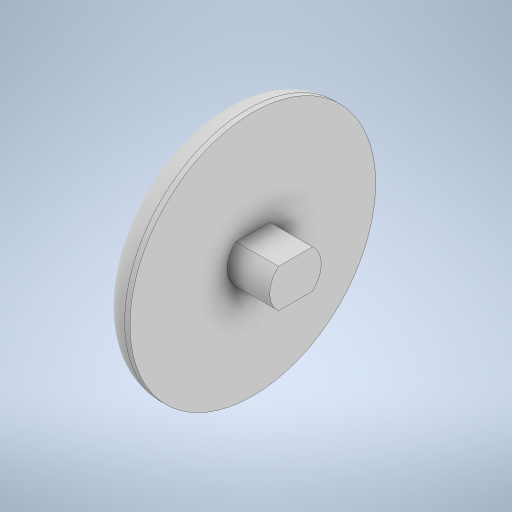
# Autodesk Inventor part: cap
Saved by Autodesk Inventor 2023 (Build 270158000, 158)
## iProperties
Created: 2025-12-21
Part Number: cap
Material: Generic
Document SubType Name: Modeling
Designer: Justin Pascual
Density: 1 g/cm^3
Appearance: Default
Author: Justin Pascual
Autodesk Inventor part; units mm, degrees
ref_plane "YZ Plane" through (0, 0, 0) normal (1, 0, 0) x (0, 1, 0)
ref_plane "XZ Plane" through (0, 0, 0) normal (0, 1, 0) x (-1, 0, 0)
ref_plane "XY Plane" through (0, 0, 0) normal (0, 0, 1) x (1, 0, 0)
sketch "Sketch1" plane through (0, 0, 0) normal (1, 0, 0) x (0, 1, 0)
  circle A0 centre (0, 0) radius 14.605
  dimension "d0" = 29.21
  constraints: 1 centre point, 1 coincident
  measures "d0" diameter of A0
extrude "Extrusion1" add sketch "Sketch1" along normal blind 3.81
sketch "Sketch2" plane through (3.81, 0, 0) normal (1, 0, 0) x (0, 0, -1)
  circle A0 centre (0, 0) radius 3.048
  dimension "d3" = 6.096
  constraints: 1 centre point, 1 coincident
  measures "d3" diameter of A0
extrude "Extrusion2" add sketch "Sketch2" along normal blind 5.08
fillet "Fillet1" radius 3.175 1 edges at (0, -14.605, 0)
sketch "Sketch4" plane through (0, 0, 0) normal (-1, 0, 0) x (0, 0, 1)
  arc A0 (-5.6465, -0.0713) -> (-5.6554, -0.2762) centre (-3.74, -0.2569) ccw
  arc A1 (-5.6141, 0.1942) -> (-5.6465, -0.0713) centre (-0.2253, -0.5991) ccw
  arc A2 (-5.5662, 0.4727) -> (-5.6141, 0.1942) centre (0.1529, -0.6547) ccw
  arc A3 (-5.5086, 0.7215) -> (-5.5662, 0.4727) centre (-1.7406, -0.2815) ccw
  arc A4 (-5.4267, 0.9766) -> (-5.5086, 0.7215) centre (-2.9409, 0.038) ccw
  arc A5 (-5.304, 1.2751) -> (-5.4267, 0.9766) centre (-0.2248, -0.9874) ccw
  arc A6 (-5.163, 1.5684) -> (-5.304, 1.2751) centre (-0.1685, -1.0125) ccw
  arc A7 (-5.0245, 1.8082) -> (-5.163, 1.5684) centre (-2.5323, 0.209) ccw
  arc A8 (-4.869, 2.0358) -> (-5.0245, 1.8082) centre (-1.0123, -0.7664) ccw
  arc A9 (-4.676, 2.2913) -> (-4.869, 2.0358) centre (2.1392, -3.0561) ccw
  arc A10 (-4.4775, 2.535) -> (-4.676, 2.2913) centre (1.9807, -2.9319) ccw
  arc A11 (-4.3056, 2.7244) -> (-4.4775, 2.535) centre (-1.6197, 0.1159) ccw
  arc A12 (-4.1196, 2.9069) -> (-4.3056, 2.7244) centre (-0.4386, -1.0312) ccw
  arc A13 (-3.8757, 3.1295) -> (-4.1196, 2.9069) centre (5.2583, -7.1259) ccw
  arc A14 (-3.6172, 3.3542) -> (-3.8757, 3.1295) centre (5.6741, -7.5927) ccw
  arc A15 (-3.384, 3.5453) -> (-3.6172, 3.3542) centre (1.9777, -3.2377) ccw
  arc A16 (-3.1278, 3.7362) -> (-3.384, 3.5453) centre (0.0717, -0.8264) ccw
  arc A17 (-2.7957, 3.9619) -> (-3.1278, 3.7362) centre (4.7659, -7.5206) ccw
  arc A18 (-2.4462, 4.1848) -> (-2.7957, 3.9619) centre (5.0689, -7.9808) ccw
  arc A19 (-2.1334, 4.3689) -> (-2.4462, 4.1848) centre (1.9799, -2.9802) ccw
  arc A20 (-1.7942, 4.5471) -> (-2.1334, 4.3689) centre (1.421, -1.9817) ccw
  arc A21 (-1.3601, 4.7537) -> (-1.7942, 4.5471) centre (6.0902, -11.4629) ccw
  arc A22 (-0.9069, 4.9546) -> (-1.3601, 4.7537) centre (6.3782, -12.0897) ccw
  arc A23 (-0.5051, 5.1169) -> (-0.9069, 4.9546) centre (3.3555, -5.0178) ccw
  arc A24 (-0.5051, 5.1169) -> (-0.1633, 5.2508) centre (-7.5686, 23.6598) ccw
  arc A25 (-0.1633, 5.2508) -> (0.1029, 5.3637) centre (-3.0503, 12.4277) ccw
  arc A26 (0.1029, 5.3637) -> (0.2863, 5.4497) centre (-2.0951, 10.2878) ccw
  arc A27 (0.2863, 5.4497) -> (0.2822, 5.4684) centre (0.282, 5.4585) ccw
  arc A28 (1.732, 5.7393) -> (1.7288, 5.6986) centre (1.7542, 5.7171) ccw
  arc A29 (1.7288, 5.6986) -> (1.8415, 5.5509) centre (5.1977, 8.2289) ccw
  arc A30 (1.8415, 5.5509) -> (1.9924, 5.3743) centre (4.5398, 7.7039) ccw
  arc A31 (1.9924, 5.3743) -> (2.1821, 5.1752) centre (6.9782, 9.9337) ccw
  arc A32 (2.4175, 4.9127) -> (2.1821, 5.1752) centre (-0.2932, 2.7193) ccw
  arc A33 (2.6207, 4.6321) -> (2.4175, 4.9127) centre (-0.1096, 2.8679) ccw
  arc A34 (2.791, 4.3346) -> (2.6207, 4.6321) centre (-0.0502, 2.9062) ccw
  arc A35 (2.9276, 4.0215) -> (2.791, 4.3346) centre (-0.0136, 2.9247) ccw
  arc A36 (3.0322, 3.7206) -> (2.9276, 4.0215) centre (-3.7608, 1.5272) ccw
  arc A37 (3.1484, 3.3453) -> (3.0322, 3.7206) centre (-12.5502, -1.3107) ccw
  arc A38 (3.2578, 2.9596) -> (3.1484, 3.3453) centre (-12.9445, -1.4276) ccw
  arc A39 (3.3418, 2.6247) -> (3.2578, 2.9596) centre (-5.6824, 0.5388) ccw
  arc A40 (3.4241, 2.1569) -> (3.3418, 2.6247) centre (-1.0267, 1.615) ccw
  arc A41 (3.4758, 1.5875) -> (3.4241, 2.1569) centre (-5.844, 1.0284) ccw
  arc A42 (3.5034, 0.8484) -> (3.4758, 1.5875) centre (-12.8805, 0.6063) ccw
  arc A43 (3.5094, -0.1688) -> (3.5034, 0.8484) centre (-53.4811, 0.0065) ccw
  arc A44 (3.4966, -1.3751) -> (3.5094, -0.1688) centre (-76.6004, 0.0774) ccw
  arc A45 (3.459, -2.053) -> (3.4966, -1.3751) centre (-5.6132, -1.2099) ccw
  arc A46 (3.3775, -2.6038) -> (3.459, -2.053) centre (-1.657, -1.5776) ccw
  arc A47 (3.2212, -3.2698) -> (3.3775, -2.6038) centre (-7.9955, -0.2856) ccw
  arc A48 (3.093, -3.71) -> (3.2212, -3.2698) centre (-6.2812, -0.7417) ccw
  arc A49 (2.941, -4.1565) -> (3.093, -3.71) centre (-7.3983, -0.3879) ccw
  arc A50 (2.7884, -4.5487) -> (2.941, -4.1565) centre (-6.23, -0.8138) ccw
  arc A51 (2.6634, -4.8003) -> (2.7884, -4.5487) centre (0.8989, -3.7662) ccw
  arc A52 (2.5346, -4.9925) -> (2.6634, -4.8003) centre (1.0054, -3.8286) ccw
  arc A53 (2.3759, -5.1807) -> (2.5346, -4.9925) centre (0.576, -3.5018) ccw
  arc A54 (2.2126, -5.3386) -> (2.3759, -5.1807) centre (0.7613, -3.6747) ccw
  arc A55 (2.0722, -5.4341) -> (2.2126, -5.3386) centre (1.7464, -4.8041) ccw
  arc A56 (1.8649, -5.5155) -> (2.0722, -5.4341) centre (1.5744, -4.4716) ccw
  arc A57 (1.6748, -5.5367) -> (1.8649, -5.5155) centre (1.7045, -4.939) ccw
  arc A58 (1.419, -5.5007) -> (1.6748, -5.5367) centre (1.746, -4.103) ccw
  arc A59 (0.9213, -5.3769) -> (1.419, -5.5007) centre (5.6118, 12.4168) ccw
  arc A60 (0.5621, -5.28) -> (0.9213, -5.3769) centre (9.1798, 25.9517) ccw
  arc A61 (0.1735, -5.1709) -> (0.5621, -5.28) centre (12.4982, 37.9783) ccw
  arc A62 (-0.1873, -5.0661) -> (0.1735, -5.1709) centre (11.5162, 34.5399) ccw
  arc A63 (-0.4514, -4.9848) -> (-0.1873, -5.0661) centre (3.3268, 6.8259) ccw
  arc A64 (-0.7227, -4.8868) -> (-0.4514, -4.9848) centre (0.738, -1.2668) ccw
  arc A65 (-1.1143, -4.7232) -> (-0.7227, -4.8868) centre (5.8148, 11.3157) ccw
  arc A66 (-1.5449, -4.531) -> (-1.1143, -4.7232) centre (6.6251, 13.1912) ccw
  arc A67 (-1.9539, -4.3357) -> (-1.5449, -4.531) centre (5.4282, 10.5949) ccw
  arc A68 (-2.372, -4.1184) -> (-1.9539, -4.3357) centre (3.2302, 6.1494) ccw
  arc A69 (-2.8306, -3.8595) -> (-2.372, -4.1184) centre (6.3574, 11.881) ccw
  arc A70 (-3.2602, -3.6002) -> (-2.8306, -3.8595) centre (5.8348, 10.9857) ccw
  arc A71 (-3.5828, -3.3849) -> (-3.2602, -3.6002) centre (0.0383, 1.6898) ccw
  arc A72 (-3.873, -3.1625) -> (-3.5828, -3.3849) centre (-0.4693, 0.9784) ccw
  arc A73 (-4.197, -2.8843) -> (-3.873, -3.1625) centre (2.4433, 4.5218) ccw
  arc A74 (-4.5043, -2.5966) -> (-4.197, -2.8843) centre (2.3234, 4.388) ccw
  arc A75 (-4.7417, -2.3458) -> (-4.5043, -2.5966) centre (-1.3894, 0.5899) ccw
  arc A76 (-4.9465, -2.0901) -> (-4.7417, -2.3458) centre (-1.9464, 0.1021) ccw
  arc A77 (-5.1523, -1.7887) -> (-4.9465, -2.0901) centre (-0.3352, 1.2794) ccw
  arc A78 (-5.3296, -1.4893) -> (-5.1523, -1.7887) centre (-0.6214, 1.0972) ccw
  arc A79 (-5.444, -1.2432) -> (-5.3296, -1.4893) centre (-3.5575, -0.5158) ccw
  arc A80 (-5.5236, -1.0061) -> (-5.444, -1.2432) centre (-2.7878, -0.2191) ccw
  arc A81 (-5.5915, -0.7375) -> (-5.5236, -1.0061) centre (-1.4164, 0.1755) ccw
  arc A82 (-5.6392, -0.479) -> (-5.5915, -0.7375) centre (-1.6866, 0.1164) ccw
  arc A83 (-5.6554, -0.2762) -> (-5.6392, -0.479) centre (-4.1953, -0.2615) ccw
  arc A84 (-0.8061, 0.9371) -> (-0.8024, 0.86) centre (-0.6453, 0.9061) ccw
  arc A85 (-0.8024, 0.86) -> (-0.7642, 0.7759) centre (-0.4887, 0.952) ccw
  arc A86 (-0.7642, 0.7759) -> (-0.6987, 0.6978) centre (-0.4301, 0.9895) ccw
  arc A87 (-0.6987, 0.6978) -> (-0.6152, 0.6385) centre (-0.4234, 0.9967) ccw
  arc A88 (-0.6152, 0.6385) -> (-0.5006, 0.591) centre (-0.3178, 1.1941) ccw
  arc A89 (-0.5006, 0.591) -> (-0.3373, 0.5486) centre (0.1071, 2.5958) ccw
  arc A90 (-0.3373, 0.5486) -> (-0.1569, 0.5168) centre (0.1561, 2.8218) ccw
  arc A91 (-0.1569, 0.5168) -> (0.0144, 0.5018) centre (0.0865, 2.3088) ccw
  arc A92 (0.0144, 0.5018) -> (0.1943, 0.5059) centre (0.0714, 1.9317) ccw
  arc A93 (0.1943, 0.5059) -> (0.401, 0.5323) centre (-0.0258, 3.0602) ccw
  arc A94 (0.401, 0.5323) -> (0.6017, 0.5747) centre (-0.017, 3.0079) ccw
  arc A95 (0.6017, 0.5747) -> (0.7626, 0.6281) centre (0.3107, 1.7191) ccw
  arc A96 (0.7626, 0.6281) -> (0.8943, 0.6933) centre (0.3445, 1.6375) ccw
  arc A97 (0.8943, 0.6933) -> (1.0055, 0.7714) centre (0.4905, 1.3868) ccw
  arc A98 (1.0055, 0.7714) -> (1.0832, 0.8503) centre (0.6344, 1.2148) ccw
  arc A99 (1.0832, 0.8503) -> (1.1065, 0.9159) centre (1.0024, 0.9159) ccw
  arc A100 (1.1065, 0.9159) -> (1.0851, 0.983) centre (0.9908, 0.9159) ccw
  arc A101 (1.0851, 0.983) -> (1.0134, 1.0668) centre (0.5836, 0.6263) ccw
  arc A102 (1.0134, 1.0668) -> (0.9109, 1.1518) centre (0.4374, 0.4764) ccw
  arc A103 (0.9109, 1.1518) -> (0.7895, 1.2252) centre (0.3037, 0.2856) ccw
  arc A104 (0.7895, 1.2252) -> (0.6424, 1.2879) centre (0.2947, 0.2683) ccw
  arc A105 (0.6424, 1.2879) -> (0.4615, 1.3405) centre (-0.0227, -0.6623) ccw
  arc A106 (0.4615, 1.3405) -> (0.2768, 1.3763) centre (-0.0219, -0.659) ccw
  arc A107 (0.2768, 1.3763) -> (0.118, 1.3876) centre (0.1228, 0.3266) ccw
  arc A108 (0.118, 1.3876) -> (-0.0373, 1.3771) centre (0.1236, 0.148) ccw
  arc A109 (-0.0373, 1.3771) -> (-0.211, 1.3467) centre (0.227, -0.6422) ccw
  arc A110 (-0.211, 1.3467) -> (-0.3762, 1.3026) centre (0.2088, -0.5599) ccw
  arc A111 (-0.3762, 1.3026) -> (-0.5042, 1.2506) centre (-0.1235, 0.4982) ccw
  arc A112 (-0.5042, 1.2506) -> (-0.6091, 1.1856) centre (-0.1798, 0.6096) ccw
  arc A113 (-0.6091, 1.1856) -> (-0.7033, 1.1026) centre (-0.1505, 0.5703) ccw
  arc A114 (-0.7033, 1.1026) -> (-0.774, 1.015) centre (-0.2392, 0.6557) ccw
  arc A115 (-0.774, 1.015) -> (-0.8061, 0.9371) centre (-0.5985, 0.8971) ccw
  arc A116 (-0.702, 0.9022) -> (-0.72, 0.8615) centre (-0.665, 0.8615) ccw
  arc A117 (-0.6411, 0.9476) -> (-0.702, 0.9022) centre (-0.4441, 0.6193) ccw
  arc A118 (-0.5542, 0.99) -> (-0.6411, 0.9476) centre (-0.35, 0.4625) ccw
  arc A119 (-0.4514, 1.0227) -> (-0.5542, 0.99) centre (-0.2383, 0.1739) ccw
  arc A120 (-0.329, 1.0437) -> (-0.4514, 1.0227) centre (-0.2529, 0.2319) ccw
  arc A121 (-0.1828, 1.0505) -> (-0.329, 1.0437) centre (-0.1828, -0.5159) ccw
  arc A122 (-0.0365, 1.0437) -> (-0.1828, 1.0505) centre (-0.1828, -0.5159) ccw
  arc A123 (0.0858, 1.0227) -> (-0.0365, 1.0437) centre (-0.1127, 0.2319) ccw
  arc A124 (0.1887, 0.99) -> (0.0858, 1.0227) centre (-0.1272, 0.1739) ccw
  arc A125 (0.2755, 0.9476) -> (0.1887, 0.99) centre (-0.0155, 0.4625) ccw
  arc A126 (0.3365, 0.9022) -> (0.2755, 0.9476) centre (0.0786, 0.6193) ccw
  arc A127 (0.3544, 0.8615) -> (0.3365, 0.9022) centre (0.2994, 0.8615) ccw
  arc A128 (0.3365, 0.8209) -> (0.3544, 0.8615) centre (0.2994, 0.8615) ccw
  arc A129 (0.2755, 0.7755) -> (0.3365, 0.8209) centre (0.0786, 1.1038) ccw
  arc A130 (0.1887, 0.7331) -> (0.2755, 0.7755) centre (-0.0155, 1.2606) ccw
  arc A131 (0.0858, 0.7004) -> (0.1887, 0.7331) centre (-0.1272, 1.5491) ccw
  arc A132 (-0.0365, 0.6794) -> (0.0858, 0.7004) centre (-0.1127, 1.4912) ccw
  arc A133 (-0.1828, 0.6726) -> (-0.0365, 0.6794) centre (-0.1828, 2.2389) ccw
  arc A134 (-0.329, 0.6794) -> (-0.1828, 0.6726) centre (-0.1828, 2.2389) ccw
  arc A135 (-0.4514, 0.7004) -> (-0.329, 0.6794) centre (-0.2529, 1.4912) ccw
  arc A136 (-0.5542, 0.7331) -> (-0.4514, 0.7004) centre (-0.2384, 1.5491) ccw
  arc A137 (-0.6411, 0.7755) -> (-0.5542, 0.7331) centre (-0.35, 1.2606) ccw
  arc A138 (-0.702, 0.8209) -> (-0.6411, 0.7755) centre (-0.4441, 1.1038) ccw
  arc A139 (-0.72, 0.8615) -> (-0.702, 0.8209) centre (-0.665, 0.8615) ccw
  arc A140 (1.1654, 2.4636) -> (1.1531, 2.1926) centre (3.902, 2.2035) ccw
  arc A141 (1.1531, 2.1926) -> (1.1654, 1.8953) centre (5.1247, 2.2083) ccw
  arc A142 (1.1654, 1.8953) -> (1.1993, 1.6066) centre (4.9828, 2.1971) ccw
  arc A143 (1.1993, 1.6066) -> (1.2524, 1.3622) centre (3.2813, 1.9315) ccw
  arc A144 (1.2524, 1.3622) -> (1.3214, 1.1513) centre (3.7833, 2.0724) ccw
  arc A145 (1.3214, 1.1513) -> (1.41, 0.9394) centre (4.14, 2.2059) ccw
  arc A146 (1.41, 0.9394) -> (1.504, 0.7559) centre (3.8105, 2.053) ccw
  arc A147 (1.504, 0.7559) -> (1.5876, 0.6397) centre (2.0638, 1.0707) ccw
  arc A148 (1.5876, 0.6397) -> (1.6762, 0.5537) centre (2.2968, 1.2815) ccw
  arc A149 (1.6762, 0.5537) -> (1.7836, 0.4708) centre (2.5832, 1.6174) ccw
  arc A150 (1.7836, 0.4708) -> (1.8928, 0.4024) centre (2.5272, 1.5371) ccw
  arc A151 (1.8928, 0.4024) -> (1.9855, 0.3623) centre (2.1366, 0.8385) ccw
  arc A152 (1.9855, 0.3623) -> (2.0826, 0.3491) centre (2.072, 0.6348) ccw
  arc A153 (2.0826, 0.3491) -> (2.2048, 0.3645) centre (2.0567, 1.0462) ccw
  arc A154 (2.2048, 0.3645) -> (2.3315, 0.4035) centre (2.0379, 1.1326) ccw
  arc A155 (2.3315, 0.4035) -> (2.4429, 0.4617) centre (2.0932, 0.9953) ccw
  arc A156 (2.4429, 0.4617) -> (2.5515, 0.5599) centre (2.1836, 0.8575) ccw
  arc A157 (2.5515, 0.5599) -> (2.6713, 0.7272) centre (1.1834, 1.6661) ccw
  arc A158 (2.6713, 0.7272) -> (2.7826, 0.9278) centre (0.9458, 1.8161) ccw
  arc A159 (2.7826, 0.9278) -> (2.8674, 1.1344) centre (1.1347, 1.7247) ccw
  arc A160 (2.8674, 1.1344) -> (2.9338, 1.3723) centre (0.7866, 1.8433) ccw
  arc A161 (2.9338, 1.3723) -> (2.9896, 1.6702) centre (-1.8893, 2.4304) ccw
  arc A162 (2.9896, 1.6702) -> (3.0279, 1.9773) centre (-2.0236, 2.4514) ccw
  arc A163 (3.0279, 1.9773) -> (3.0405, 2.2451) centre (0.1745, 2.2451) ccw
  arc A164 (3.0405, 2.2451) -> (3.0258, 2.5429) centre (0.0074, 2.2451) ccw
  arc A165 (3.0258, 2.5429) -> (2.9818, 2.8162) centre (0.7805, 2.3213) ccw
  arc A166 (2.9818, 2.8162) -> (2.9066, 3.0728) centre (0.9388, 2.3569) ccw
  arc A167 (2.9066, 3.0728) -> (2.7987, 3.3204) centre (0.8572, 2.3272) ccw
  arc A168 (2.7987, 3.3204) -> (2.6928, 3.5094) centre (0.2659, 2.0248) ccw
  arc A169 (2.6928, 3.5094) -> (2.5744, 3.6865) centre (0.4245, 2.1217) ccw
  arc A170 (2.5744, 3.6865) -> (2.4606, 3.8304) centre (0.7326, 2.346) ccw
  arc A171 (2.4606, 3.8304) -> (2.3746, 3.9031) centre (2.1908, 3.5987) ccw
  arc A172 (2.3746, 3.9031) -> (2.2771, 3.9441) centre (2.1862, 3.5911) ccw
  arc A173 (2.2771, 3.9441) -> (2.1648, 3.9591) centre (2.1579, 3.4811) ccw
  arc A174 (2.1648, 3.9591) -> (2.0389, 3.9477) centre (2.1561, 3.355) ccw
  arc A175 (2.0389, 3.9477) -> (1.9013, 3.9099) centre (2.2286, 2.9881) ccw
  arc A176 (1.9013, 3.9099) -> (1.7746, 3.8431) centre (2.0686, 3.4386) ccw
  arc A177 (1.7746, 3.8431) -> (1.6383, 3.7275) centre (2.4729, 2.8824) ccw
  arc A178 (1.6383, 3.7275) -> (1.5124, 3.5837) centre (2.568, 2.7861) ccw
  arc A179 (1.5124, 3.5837) -> (1.4159, 3.4306) centre (2.3632, 2.9409) ccw
  arc A180 (1.4159, 3.4306) -> (1.3373, 3.2447) centre (2.5829, 2.8273) ccw
  arc A181 (1.3373, 3.2447) -> (1.2621, 2.9914) centre (4.9275, 2.0417) ccw
  arc A182 (1.2621, 2.9914) -> (1.2011, 2.7174) centre (5.2222, 1.9653) ccw
  arc A183 (1.2011, 2.7174) -> (1.1654, 2.4636) centre (3.9974, 2.1944) ccw
  arc A184 (1.2182, 2.3502) -> (1.214, 2.2129) centre (3.4297, 2.2129) ccw
  arc A185 (1.2313, 2.4658) -> (1.2182, 2.3502) centre (2.364, 2.279) ccw
  arc A186 (1.2499, 2.5531) -> (1.2313, 2.4658) centre (2.1922, 2.3074) ccw
  arc A187 (1.273, 2.571) -> (1.2499, 2.5531) centre (1.273, 2.5471) ccw
  arc A188 (1.3103, 2.5638) -> (1.273, 2.571) centre (1.273, 2.4713) ccw
  arc A189 (1.4079, 2.5229) -> (1.3103, 2.5638) centre (-0.1186, -0.979) ccw
  arc A190 (1.5234, 2.4699) -> (1.4079, 2.5229) centre (0.0725, -0.5406) ccw
  arc A191 (1.6491, 2.4071) -> (1.5234, 2.4699) centre (-0.6443, -2.0277) ccw
  arc A192 (1.7704, 2.3386) -> (1.6491, 2.4071) centre (0.7674, 0.7022) ccw
  arc A193 (1.8727, 2.2685) -> (1.7704, 2.3386) centre (1.139, 1.3083) ccw
  arc A194 (1.9485, 2.2046) -> (1.8727, 2.2685) centre (1.2448, 1.4468) ccw
  arc A195 (1.9654, 2.1653) -> (1.9485, 2.2046) centre (1.9124, 2.1658) ccw
  arc A196 (1.9483, 2.1254) -> (1.9654, 2.1653) centre (1.9089, 2.1658) ccw
  arc A197 (1.8728, 2.058) -> (1.9483, 2.1254) centre (1.1542, 2.9393) ccw
  arc A198 (1.7714, 1.9832) -> (1.8728, 2.058) centre (1.0535, 3.0629) ccw
  arc A199 (1.6513, 1.9092) -> (1.7714, 1.9832) centre (0.6483, 3.6722) ccw
  arc A200 (1.5267, 1.8454) -> (1.6513, 1.9092) centre (0.8629, 3.295) ccw
  arc A201 (1.4117, 1.8015) -> (1.5267, 1.8454) centre (1.1283, 2.7154) ccw
  arc A202 (1.3184, 1.7792) -> (1.4117, 1.8015) centre (1.1989, 2.4876) ccw
  arc A203 (1.2759, 1.7928) -> (1.3184, 1.7792) centre (1.3103, 1.8272) ccw
  arc A204 (1.2517, 1.8367) -> (1.2759, 1.7928) centre (1.3396, 1.8565) ccw
  arc A205 (1.2322, 1.9417) -> (1.2517, 1.8367) centre (2.6334, 2.1483) ccw
  arc A206 (1.2185, 2.0712) -> (1.2322, 1.9417) centre (2.7946, 2.1721) ccw
  arc A207 (1.214, 2.2129) -> (1.2185, 2.0712) centre (3.4321, 2.2129) ccw
  arc A208 (1.3479, 1.4473) -> (1.3282, 1.416) centre (1.3588, 1.4186) ccw
  arc A209 (1.4339, 1.4729) -> (1.3479, 1.4473) centre (1.5622, 0.8849) ccw
  arc A210 (1.5538, 1.4908) -> (1.4339, 1.4729) centre (1.6269, 0.5885) ccw
  arc A211 (1.6975, 1.4966) -> (1.5538, 1.4908) centre (1.6975, -0.2825) ccw
  arc A212 (1.8532, 1.4879) -> (1.6975, 1.4966) centre (1.6975, 0.1) ccw
  arc A213 (1.9712, 1.4604) -> (1.8532, 1.4879) centre (1.7954, 0.973) ccw
  arc A214 (2.0452, 1.4176) -> (1.9712, 1.4604) centre (1.8895, 1.2339) ccw
  arc A215 (2.0699, 1.3623) -> (2.0452, 1.4176) centre (1.9999, 1.3642) ccw
  arc A216 (2.0548, 1.2939) -> (2.0699, 1.3623) centre (1.8855, 1.3672) ccw
  arc A217 (2.0045, 1.192) -> (2.0548, 1.2939) centre (0.9985, 1.7514) ccw
  arc A218 (1.9345, 1.0793) -> (2.0045, 1.192) centre (0.8064, 1.8582) ccw
  arc A219 (1.8524, 0.971) -> (1.9345, 1.0793) centre (0.6931, 1.9365) ccw
  arc A220 (1.767, 0.8758) -> (1.8524, 0.971) centre (0.5068, 2.0916) ccw
  arc A221 (1.6877, 0.8031) -> (1.767, 0.8758) centre (1.1305, 1.4899) ccw
  arc A222 (1.6223, 0.7566) -> (1.6877, 0.8031) centre (1.2912, 1.2918) ccw
  arc A223 (1.5923, 0.7601) -> (1.6223, 0.7566) centre (1.6095, 0.7773) ccw
  arc A224 (1.5689, 0.7918) -> (1.5923, 0.7601) centre (1.6869, 0.8547) ccw
  arc A225 (1.5288, 0.8703) -> (1.5689, 0.7918) centre (3.7941, 1.9761) ccw
  arc A226 (1.4845, 0.966) -> (1.5288, 0.8703) centre (3.8278, 1.9926) ccw
  arc A227 (1.4407, 1.0708) -> (1.4845, 0.966) centre (4.6256, 2.3421) ccw
  arc A228 (1.3997, 1.178) -> (1.4407, 1.0708) centre (4.9842, 2.4853) ccw
  arc A229 (1.3641, 1.2814) -> (1.3997, 1.178) centre (4.3502, 2.254) ccw
  arc A230 (1.3368, 1.3697) -> (1.3641, 1.2814) centre (4.14, 2.1856) ccw
  arc A231 (1.3282, 1.416) -> (1.3368, 1.3697) centre (1.5646, 1.436) ccw
  arc A232 (1.4946, 3.3391) -> (1.445, 3.2157) centre (2.7811, 2.7499) ccw
  arc A233 (1.551, 3.4433) -> (1.4946, 3.3391) centre (2.3051, 2.9679) ccw
  arc A234 (1.6061, 3.5185) -> (1.551, 3.4433) centre (2.1144, 3.0881) ccw
  arc A235 (1.6482, 3.538) -> (1.6061, 3.5185) centre (1.6482, 3.4829) ccw
  arc A236 (1.6936, 3.5234) -> (1.6482, 3.538) centre (1.6482, 3.46) ccw
  arc A237 (1.761, 3.4685) -> (1.6936, 3.5234) centre (1.2818, 2.9488) ccw
  arc A238 (1.8345, 3.3921) -> (1.761, 3.4685) centre (1.1591, 2.8158) ccw
  arc A239 (1.9046, 3.3016) -> (1.8345, 3.3921) centre (0.9213, 2.6128) ccw
  arc A240 (1.9815, 3.1794) -> (1.9046, 3.3016) centre (0.7009, 2.4585) ccw
  arc A241 (2.0077, 3.097) -> (1.9815, 3.1794) centre (1.7968, 3.0754) ccw
  arc A242 (1.9923, 3.0347) -> (2.0077, 3.097) centre (1.9128, 3.0873) ccw
  arc A243 (1.9375, 2.9809) -> (1.9923, 3.0347) centre (1.8389, 3.1362) ccw
  arc A244 (1.8701, 2.9484) -> (1.9375, 2.9809) centre (1.7658, 3.2512) ccw
  arc A245 (1.7745, 2.9209) -> (1.8701, 2.9484) centre (1.5547, 3.8647) ccw
  arc A246 (1.6689, 2.9018) -> (1.7745, 2.9209) centre (1.5307, 3.9677) ccw
  arc A247 (1.5687, 2.895) -> (1.6689, 2.9018) centre (1.563, 3.7184) ccw
  arc A248 (1.4366, 2.9046) -> (1.5687, 2.895) centre (1.563, 3.7246) ccw
  arc A249 (1.3874, 2.9443) -> (1.4366, 2.9046) centre (1.4462, 2.967) ccw
  arc A250 (1.3838, 3.0228) -> (1.3874, 2.9443) centre (1.5028, 2.9888) ccw
  arc A251 (1.445, 3.2157) -> (1.3838, 3.0228) centre (4.7919, 2.0489) ccw
  arc A252 (2.1972, 1.7411) -> (2.1809, 1.7111) centre (2.2168, 1.7111) ccw
  arc A253 (2.2814, 1.7919) -> (2.1972, 1.7411) centre (2.9447, 0.5967) ccw
  arc A254 (2.392, 1.8471) -> (2.2814, 1.7919) centre (2.966, 0.5583) ccw
  arc A255 (2.523, 1.9009) -> (2.392, 1.8471) centre (3.384, -0.3801) ccw
  arc A256 (2.6573, 1.9472) -> (2.523, 1.9009) centre (3.385, -0.3827) ccw
  arc A257 (2.7776, 1.9792) -> (2.6573, 1.9472) centre (3.0878, 0.5689) ccw
  arc A258 (2.8756, 1.9971) -> (2.7776, 1.9792) centre (3.0786, 0.6109) ccw
  arc A259 (2.9093, 1.9859) -> (2.8756, 1.9971) centre (2.8813, 1.9579) ccw
  arc A260 (2.9231, 1.9523) -> (2.9093, 1.9859) centre (2.8761, 1.9526) ccw
  arc A261 (2.9192, 1.8575) -> (2.9231, 1.9523) centre (1.5449, 1.962) ccw
  arc A262 (2.9054, 1.7408) -> (2.9192, 1.8575) centre (1.4976, 1.9656) ccw
  arc A263 (2.8808, 1.6108) -> (2.9054, 1.7408) centre (0.6483, 2.1011) ccw
  line L0 (2.8808, 1.6108) -> (2.8081, 1.2799)
  line L1 (2.8081, 1.2799) -> (2.4945, 1.4651)
  arc A264 (2.3744, 1.5405) -> (2.4945, 1.4651) centre (3.8412, 3.7449) ccw
  arc A265 (2.2731, 1.6138) -> (2.3744, 1.5405) centre (3.2629, 2.8758) ccw
  arc A266 (2.1955, 1.6786) -> (2.2731, 1.6138) centre (3.281, 2.8988) ccw
  arc A267 (2.1809, 1.7111) -> (2.1955, 1.6786) centre (2.2245, 1.7111) ccw
  arc A268 (2.4915, 2.9875) -> (2.3929, 2.9125) centre (3.6417, 1.3703) ccw
  arc A269 (2.5882, 3.0507) -> (2.4915, 2.9875) centre (3.3613, 1.7646) ccw
  arc A270 (2.672, 3.0971) -> (2.5882, 3.0507) centre (3.276, 1.9064) ccw
  arc A271 (2.7184, 3.1082) -> (2.672, 3.0971) centre (2.7184, 3.0057) ccw
  arc A272 (2.7553, 3.0904) -> (2.7184, 3.1082) centre (2.7184, 3.0611) ccw
  arc A273 (2.7984, 3.0256) -> (2.7553, 3.0904) centre (2.3934, 2.8032) ccw
  arc A274 (2.8397, 2.9347) -> (2.7984, 3.0256) centre (2.218, 2.7068) ccw
  arc A275 (2.8729, 2.8269) -> (2.8397, 2.9347) centre (1.8348, 2.5664) ccw
  arc A276 (2.8959, 2.7152) -> (2.8729, 2.8269) centre (1.5907, 2.5051) ccw
  arc A277 (2.9065, 2.612) -> (2.8959, 2.7152) centre (2.0031, 2.5715) ccw
  arc A278 (2.9054, 2.5283) -> (2.9065, 2.612) centre (2.1785, 2.5794) ccw
  arc A279 (2.888, 2.4902) -> (2.9054, 2.5283) centre (2.8456, 2.5325) ccw
  arc A280 (2.8479, 2.4761) -> (2.888, 2.4902) centre (2.8534, 2.5248) ccw
  arc A281 (2.7487, 2.4924) -> (2.8479, 2.4761) centre (2.9609, 3.4746) ccw
  arc A282 (2.6264, 2.5257) -> (2.7487, 2.4924) centre (3.0006, 3.6583) ccw
  arc A283 (2.4918, 2.5758) -> (2.6264, 2.5257) centre (3.2389, 4.3794) ccw
  line L2 (2.4918, 2.5758) -> (2.1512, 2.7169)
  line L3 (2.1512, 2.7169) -> (2.3929, 2.9125)
  arc A284 (1.732, 5.7393) -> (0.2822, 5.4684) centre (3.3012, -6.6735) ccw
  arc A285 (-1.0633, 2.9568) -> (-1.0596, 2.8797) centre (-0.9025, 2.9258) ccw
  arc A286 (-1.0596, 2.8797) -> (-1.0214, 2.7956) centre (-0.7459, 2.9717) ccw
  arc A287 (-1.0214, 2.7956) -> (-0.9559, 2.7175) centre (-0.6873, 3.0092) ccw
  arc A288 (-0.9559, 2.7175) -> (-0.8724, 2.6582) centre (-0.6806, 3.0164) ccw
  arc A289 (-0.8724, 2.6582) -> (-0.7578, 2.6107) centre (-0.575, 3.2138) ccw
  arc A290 (-0.7578, 2.6107) -> (-0.5945, 2.5683) centre (-0.1501, 4.6155) ccw
  arc A291 (-0.5945, 2.5683) -> (-0.4141, 2.5365) centre (-0.1011, 4.8415) ccw
  arc A292 (-0.4141, 2.5365) -> (-0.2428, 2.5215) centre (-0.1707, 4.3285) ccw
  arc A293 (-0.2428, 2.5215) -> (-0.0629, 2.5256) centre (-0.1858, 3.9514) ccw
  arc A294 (-0.0629, 2.5256) -> (0.1438, 2.552) centre (-0.283, 5.0799) ccw
  arc A295 (0.1438, 2.552) -> (0.3445, 2.5944) centre (-0.2742, 5.0276) ccw
  arc A296 (0.3445, 2.5944) -> (0.5054, 2.6478) centre (0.0535, 3.7388) ccw
  arc A297 (0.5054, 2.6478) -> (0.6371, 2.713) centre (0.0873, 3.6572) ccw
  arc A298 (0.6371, 2.713) -> (0.7483, 2.7911) centre (0.2333, 3.4065) ccw
  arc A299 (0.7483, 2.7911) -> (0.826, 2.87) centre (0.3772, 3.2345) ccw
  arc A300 (0.826, 2.87) -> (0.8493, 2.9356) centre (0.7452, 2.9356) ccw
  arc A301 (0.8493, 2.9356) -> (0.8279, 3.0027) centre (0.7336, 2.9356) ccw
  arc A302 (0.8279, 3.0027) -> (0.7562, 3.0865) centre (0.3264, 2.646) ccw
  arc A303 (0.7562, 3.0865) -> (0.6537, 3.1715) centre (0.1802, 2.4961) ccw
  arc A304 (0.6537, 3.1715) -> (0.5323, 3.2449) centre (0.0465, 2.3053) ccw
  arc A305 (0.5323, 3.2449) -> (0.3852, 3.3076) centre (0.0375, 2.288) ccw
  arc A306 (0.3852, 3.3076) -> (0.2043, 3.3602) centre (-0.2799, 1.3574) ccw
  arc A307 (0.2043, 3.3602) -> (0.0196, 3.396) centre (-0.2791, 1.3607) ccw
  arc A308 (0.0196, 3.396) -> (-0.1392, 3.4073) centre (-0.1344, 2.3463) ccw
  arc A309 (-0.1392, 3.4073) -> (-0.2945, 3.3968) centre (-0.1336, 2.1677) ccw
  arc A310 (-0.2945, 3.3968) -> (-0.4682, 3.3664) centre (-0.0302, 1.3775) ccw
  arc A311 (-0.4682, 3.3664) -> (-0.6334, 3.3223) centre (-0.0484, 1.4598) ccw
  arc A312 (-0.6334, 3.3223) -> (-0.7614, 3.2703) centre (-0.3807, 2.5179) ccw
  arc A313 (-0.7614, 3.2703) -> (-0.8663, 3.2053) centre (-0.437, 2.6293) ccw
  arc A314 (-0.8663, 3.2053) -> (-0.9605, 3.1223) centre (-0.4077, 2.59) ccw
  arc A315 (-0.9605, 3.1223) -> (-1.0312, 3.0347) centre (-0.4964, 2.6754) ccw
  arc A316 (-1.0312, 3.0347) -> (-1.0633, 2.9568) centre (-0.8557, 2.9168) ccw
  arc A317 (-0.9592, 2.9219) -> (-0.9772, 2.8812) centre (-0.9222, 2.8812) ccw
  arc A318 (-0.8983, 2.9673) -> (-0.9592, 2.9219) centre (-0.7013, 2.639) ccw
  arc A319 (-0.8114, 3.0097) -> (-0.8983, 2.9673) centre (-0.6072, 2.4822) ccw
  arc A320 (-0.7086, 3.0424) -> (-0.8114, 3.0097) centre (-0.4956, 2.1936) ccw
  arc A321 (-0.5862, 3.0634) -> (-0.7086, 3.0424) centre (-0.5101, 2.2516) ccw
  arc A322 (-0.44, 3.0702) -> (-0.5862, 3.0634) centre (-0.44, 1.5038) ccw
  arc A323 (-0.2937, 3.0634) -> (-0.44, 3.0702) centre (-0.44, 1.5038) ccw
  arc A324 (-0.1714, 3.0424) -> (-0.2937, 3.0634) centre (-0.3699, 2.2516) ccw
  arc A325 (-0.0685, 3.0097) -> (-0.1714, 3.0424) centre (-0.3844, 2.1936) ccw
  arc A326 (0.0183, 2.9673) -> (-0.0685, 3.0097) centre (-0.2727, 2.4822) ccw
  arc A327 (0.0793, 2.9219) -> (0.0183, 2.9673) centre (-0.1786, 2.639) ccw
  arc A328 (0.0972, 2.8812) -> (0.0793, 2.9219) centre (0.0422, 2.8812) ccw
  arc A329 (0.0793, 2.8406) -> (0.0972, 2.8812) centre (0.0422, 2.8812) ccw
  arc A330 (0.0183, 2.7952) -> (0.0793, 2.8406) centre (-0.1786, 3.1235) ccw
  arc A331 (-0.0685, 2.7528) -> (0.0183, 2.7952) centre (-0.2727, 3.2803) ccw
  arc A332 (-0.1714, 2.7201) -> (-0.0685, 2.7528) centre (-0.3844, 3.5688) ccw
  arc A333 (-0.2937, 2.6991) -> (-0.1714, 2.7201) centre (-0.3699, 3.5109) ccw
  arc A334 (-0.44, 2.6923) -> (-0.2937, 2.6991) centre (-0.44, 4.2586) ccw
  arc A335 (-0.5862, 2.6991) -> (-0.44, 2.6923) centre (-0.44, 4.2586) ccw
  arc A336 (-0.7086, 2.7201) -> (-0.5862, 2.6991) centre (-0.5101, 3.5109) ccw
  arc A337 (-0.8114, 2.7528) -> (-0.7086, 2.7201) centre (-0.4956, 3.5688) ccw
  arc A338 (-0.8983, 2.7952) -> (-0.8114, 2.7528) centre (-0.6072, 3.2803) ccw
  arc A339 (-0.9592, 2.8406) -> (-0.8983, 2.7952) centre (-0.7013, 3.1235) ccw
  arc A340 (-0.9772, 2.8812) -> (-0.9592, 2.8406) centre (-0.9222, 2.8812) ccw
  point P0 (0, 0)
  point P1 (-0.7265, 2.9981)
  point P2 (-0.5924, 3.2991)
  point P3 (-0.8786, 3.1169)
  point P4 (0.5102, 2.7219)
  constraints: 682 point on circle, 341 centre point, 8 end point
emboss "Emboss1" sketch "Sketch4" operation add depth 0.508 direction (1, 0, 0)
sketch "Sketch5" plane through (8.89, 0, 0) normal (1, 0, 0) x (0, 0, -1)
  arc A0 (2.0264, 2.286) -> (-2.0264, 2.286) centre (0, 0) ccw
  circle A1 centre (0, 0) radius 3.048 projected
  line L0 (2.0161, 2.286) -> (-2.0161, 2.286)
  line L1 (2.0161, -2.286) -> (-2.0161, -2.286)
  arc A2 (2.0264, -2.286) -> (2.0264, 2.286) centre (0, 0) ccw construction
  arc A3 (-2.0264, -2.286) -> (2.0264, -2.286) centre (0, 0) ccw
  arc A4 (-2.0264, 2.286) -> (-2.0264, -2.286) centre (0, 0) ccw construction
  dimension "d19" = 4.572
  constraints: 12 point on circle, 4 centre point, 4 end point, 4 point on line, 2 horizontal, 1 coincident
  measures "d19" distance between parallel lines of L0 L1
extrude "Extrusion3" cut sketch "Sketch5" against normal up to surface (5.08 mm away) contours L0 A1 | A1 L1
body "Solid1"
